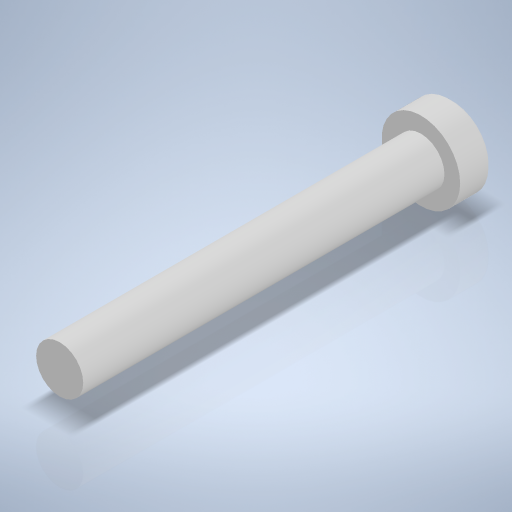
# Autodesk Inventor part: 1 part 10
Saved by Autodesk Inventor 2024 (Build 280153000, 153)
## iProperties
Created: 2024-07-24
Part Number: 1 part 10
Material: Generisch
Document SubType Name: Modeling
Designer: ffogue
Density: 1 g/cm^3
Appearance: Vorgabe
Author: ffogue
Autodesk Inventor part; units mm, degrees
ref_plane "YZ Plane" through (0, 0, 0) normal (1, 0, 0) x (0, 1, 0)
ref_plane "XZ Plane" through (0, 0, 0) normal (0, 1, 0) x (-1, 0, 0)
ref_plane "XY Plane" through (0, 0, 0) normal (0, 0, 1) x (1, 0, 0)
sketch "Skizze1" plane through (0, 0, 0) normal (0, 0, 1) x (1, 0, 0)
  line L0 (0, 0) -> (1.5, 0)
  line L1 (1.5, 0) -> (1.5, 23)
  line L2 (1.5, 23) -> (2.5, 23)
  line L3 (2.5, 23) -> (2.5, 25)
  line L4 (2.5, 25) -> (0, 25)
  line L5 (0, 25) -> (0, 0)
  dimension "d0" = 3
  dimension "d1" = 2
  dimension "d2" = 5
  dimension "d3" = 23
  constraints: 12 end point, 5 perpendicular, 1 horizontal
  measures "d0" diameter of L1 L5
  measures "d1" distance of L2.end L3.end
  measures "d2" diameter of L3 L5
  measures "d3" distance of L0.end L1.end
revolve "Umdrehung1" add sketch "Skizze1" angle 360 about axis through (0, 25, 0) along (0, -1, 0)
chamfer "Fasen1" distance 0.2 angle 45 1 edges at (-2.5, 25, 0)
